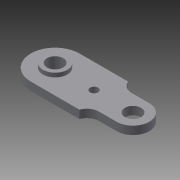
# Autodesk Inventor part: HW 5 Part 1
Saved by Autodesk Inventor 2015 SP1 (Build 190203100, 203)
## iProperties
Created: 2016-02-03
Part Number: HW 5 Part 1
Material: Generic
Document SubType Name: Modeling
Designer: melissa.roth
Density: 1 g/cm^3
Appearance: Default
Author: melissa.roth
Autodesk Inventor part; units mm, degrees
ref_plane "YZ Plane" through (0, 0, 0) normal (1, 0, 0) x (0, 1, 0)
ref_plane "XZ Plane" through (0, 0, 0) normal (0, 1, 0) x (-1, 0, 0)
ref_plane "XY Plane" through (0, 0, 0) normal (0, 0, 1) x (1, 0, 0)
sketch "Sketch1" plane through (0, 0, 0) normal (0, 0, 1) x (1, 0, 0)
  line L0 (-19.3557, 89.8434) -> (40.6443, 89.8434)
  line L1 (-19.3557, 29.8434) -> (40.6443, 29.8434)
  line L2 (54.7864, 79.8434) -> (76.6443, 79.8434)
  line L3 (54.7864, 39.8434) -> (76.6443, 39.8434)
  arc A0 (-19.3557, 89.8434) -> (-19.3557, 29.8434) centre (-19.3557, 59.8434) ccw
  arc A1 (76.6443, 39.8434) -> (76.6443, 79.8434) centre (76.6443, 59.8434) ccw
  arc A2 (54.7864, 39.8434) -> (40.6443, 29.8434) centre (54.7864, 24.8434) ccw
  arc A3 (40.6443, 89.8434) -> (54.7864, 79.8434) centre (54.7864, 94.8434) ccw
  circle A4 centre (-19.3557, 59.8434) radius 10
  circle A5 centre (28.6443, 59.8434) radius 5
  circle A6 centre (76.6443, 59.8434) radius 10
  dimension "d11" = 15
  dimension "d12" = 15
  dimension "d13" = 30
  dimension "d14" = 20
  dimension "d15" = 96
  dimension "d16" = 60
  dimension "d18" = 20
  dimension "d19" = 10
  dimension "d20" = 20
  dimension "d21" = 48
  constraints: 8 end point, 8 point on circle, 7 centre point, 6 tangent, 4 horizontal, 2 coincident, 2 parallel
  measures "d11" radius of A3
  measures "d12" radius of A2
  measures "d13" radius of A0
  measures "d14" radius of A1
  measures "d15" distance of A1.centre A0.centre
  measures "d16" horizontal distance of L0.end A0.centre
  measures "d18" diameter of A4
  measures "d19" diameter of A5
  measures "d20" diameter of A6
  measures "d21" distance of A5.centre A0.centre
extrude "Extrusion1" add sketch "Sketch1" along normal blind 10
sketch "Sketch2" plane through (0, 0, 10) normal (0, 0, 1) x (1, 0, 0)
  circle A0 centre (-19.3557, 59.8434) radius 10 projected
  circle A1 centre (-19.3557, 59.8434) radius 15
  circle A2 centre (-19.3557, 59.8434) radius 10
  point P0 (0, 0)
  dimension "d24" = 30
  dimension "d25" = 20
  constraints: 2 centre point, 2 coincident
  measures "d24" diameter of A1
  measures "d25" diameter of A2
extrude "Extrusion2" add sketch "Sketch2" along normal blind 5
equation "\"d14\" = 0.666667 * d13"
equation "\"d15\" = 2 * d21"
equation "\"d16\" = 1.25 * d21"
equation "\"d18\" = 0.666667 * d13"
equation "\"d19\" = 0.333333 * d13"
equation "\"d20\" = 0.666667 * d13"
equation "\"d24\" = d13"
equation "\"d25\" = 0.666667 * d13"
equation "\"d26\" = 0.5 * d22"
equation "\"d22\" = 10"
body "Solid1"
